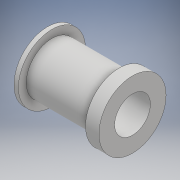
# Autodesk Inventor part: pignon 12 dents
Saved by Autodesk Inventor 2018.1 (Build 221171000, 171)
## iProperties
Created: 2022-06-30
Part Number: pignon 12 dents
Material: Generic
Document SubType Name: Modeling
Designer: mouta
Density: 1 g/cm^3
Appearance: Default
Author: mouta
Autodesk Inventor part; units mm, degrees
ref_plane "YZ Plane" through (0, 0, 0) normal (1, 0, 0) x (0, 1, 0)
ref_plane "XZ Plane" through (0, 0, 0) normal (0, 1, 0) x (-1, 0, 0)
ref_plane "XY Plane" through (0, 0, 0) normal (0, 0, 1) x (1, 0, 0)
sketch "Sketch1" plane through (0, 0, 0) normal (0, 0, 1) x (1, 0, 0)
  line L0 (0, 0) -> (4, 0)
  line L1 (0, 0) -> (0, 2.5)
  line L2 (0, 5.75) -> (15, 5.75)
  line L3 (15, 5.75) -> (15, 7.5)
  line L4 (18, 5) -> (18, 4)
  line L5 (18, 4) -> (6, 4)
  line L6 (6, 4) -> (6, 2.5)
  line L7 (6, 2.5) -> (0, 2.5)
  line L8 (0, 5.75) -> (0, 7.5)
  line L9 (0, 7.5) -> (-1, 7.5)
  line L10 (-1, 7.5) -> (-1, 2.5)
  line L11 (-1, 2.5) -> (0, 2.5)
  line L12 (15, 7.5) -> (18, 7.5)
  line L13 (18, 7.5) -> (18, 5)
  dimension "d0" = 4
  dimension "d1" = 5.75
  dimension "d2" = 15
  dimension "d3" = 1.75
  dimension "d7" = 1
  dimension "d8" = 12
  dimension "d9" = 1.5
  dimension "d11" = 1
  constraints: 28 end point, 9 perpendicular, 2 horizontal, 2 vertical
  measures "d0" distance of L0.start L0.end
  measures "d1" distance of L0.start L2.start
  measures "d2" distance of L2.start L2.end
  measures "d3" distance of L2.end L3.end
  measures "d7" distance of L4.start L4.end
  measures "d8" distance of L4.end L5.end
  measures "d9" distance of L5.end L6.end
  measures "d11" distance of L8.end L9.end
revolve "Revolution1" add sketch "Sketch1" angle 360 about axis through (0, 0, 0) along (1, 0, 0)
body "Solid1"
